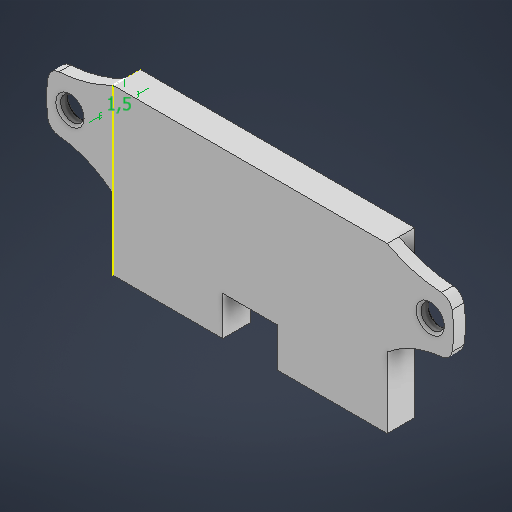
# Autodesk Inventor part: casereceiver
Saved by Autodesk Inventor 2026.1 (Build 301233000, 233)
## iProperties
Created: 2026-04-30
Part Number: casereceiver
Material: Generic
Document SubType Name: Modeling
Designer: ayjuni03
Density: 1 g/cm^3
Appearance: Default
Author: ayjuni03
Autodesk Inventor part; units mm, degrees
ref_plane "YZ Plane" through (0, 0, 0) normal (1, 0, 0) x (0, 1, 0)
ref_plane "XZ Plane" through (0, 0, 0) normal (0, 1, 0) x (-1, 0, 0)
ref_plane "XY Plane" through (0, 0, 0) normal (0, 0, 1) x (1, 0, 0)
sketch "Sketch1" plane through (0, 0, 0) normal (0, 0, 1) x (1, 0, 0)
  line L0 (0, 0) -> (-17.5, 0) construction
  line L1 (-17.5, 0) -> (17.5, 0) construction
  line L2 (17.5, 0) -> (17.5, -10.5)
  line L3 (17.5, -10.5) -> (17.5, 10.5)
  line L4 (17.5, 10.5) -> (-17.5, 10.5)
  line L5 (-17.5, 10.5) -> (-17.5, -10.5)
  line L6 (17.5, -10.5) -> (3.5, -10.5)
  line L7 (3.5, -10.5) -> (3.5, -5.5)
  line L8 (3.5, -5.5) -> (-3.5, -5.5)
  line L9 (-3.5, -5.5) -> (-3.5, -10.5)
  line L10 (-3.5, -10.5) -> (-17.5, -10.5)
  dimension "d4" = 17.5
  dimension "d5" = 35
  dimension "d6" = 10.5
  dimension "d7" = 21
  dimension "d8" = 14
  dimension "d9" = 5
  dimension "d10" = 7
  constraints: 22 end point, 7 perpendicular, 3 point on line, 1 horizontal, 1 vertical
  measures "d4" distance of L0.start L0.end
  measures "d5" distance of L0.end L1.end
  measures "d6" distance of L1.end L2.end
  measures "d7" distance of L2.end L3.end
  measures "d8" distance of L2.end L6.end
  measures "d9" distance of L6.end L7.end
  measures "d10" distance of L7.end L8.end
extrude "Extrusion1" add sketch "Sketch1" along normal blind 3.5
sketch "Sketch2" plane through (0, 0, 0) normal (0, 0, -1) x (-1, 0, 0)
  line L0 (-17.5, -10.5) -> (-17.5, 10.5) construction
  line L1 (-17.5, 10.5) -> (-16.5, 10.5) construction
  line L2 (-17.5, 10.5) -> (17.5, 10.5) construction
  line L3 (-16.5, 10.5) -> (-16.5, 9.5) construction
  line L4 (-16.5, 9.5) -> (-17.5, 9.5) construction
  line L5 (-16.5, 9.5) -> (-13.5, 9.5) construction
  line L6 (-15, 9.5) -> (-15, 8) construction
  line L7 (-16.5, 9.5) -> (-16.5, 7.1912) construction
  circle A0 centre (-15, 8) radius 1.5 construction
  circle A1 centre (-15, 8) radius 1.5
  line L8 (-15, 8) -> (-17.5, 8) construction
  line L9 (17.5, 10.5) -> (17.5, -10.5) construction
  line L10 (17.5, 10.5) -> (16.5, 10.5) construction
  line L11 (16.5, 10.5) -> (17.5, 10.5) construction
  line L12 (17.5, 10.5) -> (17.5, 9.5) construction
  line L13 (17.5, 9.5) -> (17.5, 5.455) construction
  line L14 (17.5, 10.5) -> (15, 10.5) construction
  line L15 (15, 10.5) -> (15, 8) construction
  line L16 (15, 8) -> (17.5, 8) construction
  circle A2 centre (15, 8) radius 1.5 construction
  circle A3 centre (15, 8) radius 1.5
  point P0 (0, 0)
  dimension "d13" = 1
  dimension "d14" = 1
  dimension "d15" = 3
  dimension "d16" = 1.5
  dimension "d17" = 3
  dimension "d18" = 1
  dimension "d19" = 1
  dimension "d20" = 2.5
  dimension "d21" = 2.5
  dimension "d22" = 3
  constraints: 28 end point, 8 point on line, 6 perpendicular, 4 centre point, 4 coincident, 2 concentric, 2 vertical, 1 horizontal, 1 midpoint
  measures "d13" distance of L0.end L1.end
  measures "d14" distance of L1.end L3.end
  measures "d15" distance of L3.end L5.end
  measures "d16" distance of L6.start L6.end
  measures "d17" diameter of A0
  measures "d18" distance of L2.end L10.end
  measures "d19" distance of L2.end L12.end
  measures "d20" distance of L2.end L14.end
  measures "d21" distance of L14.end L15.end
  measures "d22" diameter of A2
extrude "Extrusion2" add sketch "Sketch2" along normal blind 1
sketch "Sketch3" plane through (-17.5, -10.5, 0) normal (-1, 0, 0) x (0, 0, 1)
  line L0 (0, 21) -> (3.5, 21) construction
  line L1 (3.5, 21) -> (2, 21) construction
  line L2 (2, 21) -> (2, 0)
  line L3 (0, 0) -> (3.5, 0) projected
  line L4 (3.5, 0) -> (2, 0)
  line L5 (3.5, 21) -> (3.5, 0) projected
  line L6 (3.5, 0) -> (3.5, 21)
  line L7 (3.5, 21) -> (2, 21)
  point P0 (0, 10.5)
  dimension "d25" = 1.5
  constraints: 10 end point, 2 collinear, 2 perpendicular, 2 point on line
  measures "d25" distance of L0.end L1.end
sketch "Sketch4" plane through (0, 0, 3.5) normal (0, 0, 1) x (1, 0, 0)
  line L0 (17.5, 10.5) -> (-17.5, 10.5) projected
  line L1 (-17.5, 10.5) -> (-17.5, 8.5)
  line L2 (-17.5, 10.5) -> (-17.5, -10.5) projected
  line L3 (-17.5, 8.5) -> (-25.5, 8.5) construction
  line L4 (-17.5, 10.5) -> (-17.5, 1.5) construction
  line L5 (-17.5, 10.5) -> (-17.5, -1.5) construction
  line L6 (-17.5, -1.5) -> (-17.5, 1.5) construction
  line L7 (-17.5, 1.5) -> (-25.5542, 1.5) construction
  arc A0 (-17.5, -1.5) -> (-25.5542, 1.5) centre (-25.5542, -10.8116) ccw
  arc A1 (-25.5, 8.5) -> (-17.5, 10.5) centre (-25.5, 25.5) ccw
  line L8 (-17.5, 5) -> (-21.5, 5) construction
  line L9 (-21.5, 5) -> (-23, 5) construction
  circle A2 centre (-23, 5) radius 1.5
  line L10 (-24.5, 5) -> (-26, 5) construction
  arc A3 (-25.5, 8.5) -> (-25.5542, 1.5) centre (-12.8112, 4.9016) ccw
  line L11 (17.5, -10.5) -> (17.5, 10.5) projected
  line L12 (17.5, 10.5) -> (17.5, 8.5)
  line L13 (17.5, 10.5) -> (17.5, -1.5)
  line L14 (17.5, 10.5) -> (17.5, 8.5)
  line L15 (17.5, -1.5) -> (17.5, 1.5)
  line L16 (17.5, 8.5) -> (25.5, 8.5) construction
  line L17 (17.5, 1.5) -> (25.5, 1.5) construction
  arc A4 (25.5, 1.5) -> (17.5, -1.5) centre (25.5545, -10.8119) ccw
  arc A5 (17.5, 10.5) -> (25.5, 8.5) centre (25.5, 25.5) ccw
  line L18 (25.5, 8.5) -> (25.5, 5) construction
  line L19 (17.5, 5) -> (21.5, 5) construction
  line L20 (21.5, 5) -> (23, 5) construction
  circle A6 centre (23, 5) radius 1.5
  line L21 (24.5, 5) -> (26, 5) construction
  arc A7 (25.5, 1.5) -> (25.5, 8.5) centre (13.5, 5) ccw
  point P0 (0, 0)
  dimension "d33" = 3
  dimension "d44" = 3
  dimension "d26" = 2
  dimension "d27" = 8
  dimension "d28" = 9
  dimension "d29" = 12
  dimension "d30" = 12.3116
  dimension "d31" = 4
  dimension "d32" = 1.5
  dimension "d34" = 1.5
  dimension "d35" = 12
  dimension "d36" = 2
  dimension "d37" = 3
  dimension "d38" = 8
  dimension "d39" = 12.312
  dimension "d40" = 17
  dimension "d41" = 3.5
  dimension "d42" = 4
  dimension "d43" = 1.5
  dimension "d45" = 1.5
  constraints: 38 end point, 14 point on circle, 10 point on line, 6 centre point, 6 horizontal, 2 coincident, 2 collinear, 2 horizontal alignment, 2 perpendicular, 2 tangent, 1 vertical, 4 other
  measures "d26" distance of L0.end L1.end
  measures "d27" distance of L1.end L3.end
  measures "d28" distance of L0.end L4.end
  measures "d29" distance of L0.end L5.end
  measures "d30" radius of A0
  measures "d31" distance of L8.start L8.end
  measures "d32" distance of L8.end L9.end
  measures "d34" distance of L10.start L10.end
  measures "d35" distance of L0.start L13.end
  measures "d36" distance of L0.start L12.end
  measures "d37" distance of L13.end L15.end
  measures "d38" distance of L12.end L16.end
  measures "d39" radius of A4
  measures "d40" radius of A5
  measures "d41" distance of L16.end L18.end
  measures "d42" distance of L19.start L19.end
  measures "d43" distance of L19.end L20.end
  measures "d45" distance of L21.start L21.end
extrude "Extrusion3" add sketch "Sketch4" against normal blind 1.5
fillet "Fillet1" radius 1.5 4 edges at (-25.5, 8.5, 2.75) (-25.5542, 1.5, 2.75) (25.5, 1.5, 2.75) (25.5, 8.5, 2.75)
chamfer "Chamfer1" distance 0.3084 angle 45 1 edges at (21.5, 5, 3.5)
chamfer "Chamfer2" distance 0.3084 angle 45 3 edges at (21.5, 5, 2) (-24.5, 5, 3.5) (-24.5, 5, 2)
thread "Thread1" size "M3x0.5" class "6H" standard "ISO Metric profile" full length
thread "Thread2" size "M3x0.5" class "6H" standard "ISO Metric profile" full length
body "Solid1"
